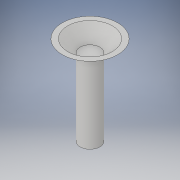
# Autodesk Inventor part: Part4
Saved by Autodesk Inventor 2018 (Build 220112000, 112)
## iProperties
Created: 2018-10-16
Part Number: Part4
Material: Generic
Document SubType Name: Modeling
Designer: Abhay
Density: 1 g/cm^3
Appearance: Default
Author: Abhay
Autodesk Inventor part; units mm, degrees
ref_plane "YZ Plane" through (0, 0, 0) normal (1, 0, 0) x (0, 1, 0)
ref_plane "XZ Plane" through (0, 0, 0) normal (0, 1, 0) x (-1, 0, 0)
ref_plane "XY Plane" through (0, 0, 0) normal (0, 0, 1) x (1, 0, 0)
sketch "Sketch1" plane through (0, 0, 0) normal (0, 0, 1) x (1, 0, 0)
  line L0 (0, 0) -> (30, 0)
  line L1 (0, -96.3621) -> (0, 0)
  line L2 (30, 0) -> (10.6955, -13.2267)
  line L3 (10.6955, -13.2267) -> (10.6955, -96.3621)
  line L4 (10.6955, -96.3621) -> (0, -96.3621)
  dimension "d0" = 30
  constraints: 10 end point, 2 horizontal
  measures "d0" distance of L0.start L0.end
revolve "Revolution1" add sketch "Sketch1" angle 360 about axis through (0, -96.3621, 0) along (0, 1, 0)
sketch "Sketch3" plane through (0, 0, 0) normal (0, 1, 0) x (1, 0, 0)
  circle A0 centre (0, 0) radius 24.25
  dimension "d8" = 48.5
  constraints: 1 centre point, 1 coincident
  measures "d8" diameter of A0
loft "Loft2" cut profiles "Sketch3" section 2 edges at (-10.6955, -13.2267, 0)
body "Solid1"
